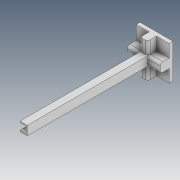
# Autodesk Inventor part: suporte para arma
Saved by Autodesk Inventor 2021 (Build 250183000, 183)
## iProperties
Created: 2020-10-22
Part Number: suporte para arma
Material: Genérico
Document SubType Name: Modeling
Designer: evert
Density: 1 g/cm^3
Appearance: Padrão
Author: evert
Autodesk Inventor part; units mm, degrees
ref_plane "YZ Plane" through (0, 0, 0) normal (1, 0, 0) x (0, 1, 0)
ref_plane "XZ Plane" through (0, 0, 0) normal (0, 1, 0) x (-1, 0, 0)
ref_plane "XY Plane" through (0, 0, 0) normal (0, 0, 1) x (1, 0, 0)
sketch "Esboço1" plane through (0, 0, 0) normal (0, 0, 1) x (1, 0, 0)
  point P0 (0, 0)
sketch "Esboço2" plane through (0, 0, 0) normal (0, 0, 1) x (1, 0, 0)
  line L0 (0, 0) -> (0, 7.2)
  line L1 (0, 7.2) -> (-5.75, 7.2)
  line L2 (-5.75, 7.2) -> (-5.75, 6.2)
  line L3 (-5.75, 6.2) -> (-1, 6.2)
  line L4 (-1, 6.2) -> (-1, 1)
  line L5 (0, 0) -> (-5.75, 0)
  line L6 (-5.75, 0) -> (-5.75, 1)
  line L7 (-5.75, 1) -> (-1, 1)
  dimension "d0" = 7.2
  dimension "d1" = 1
  dimension "d2" = 5.75
  dimension "d3" = 4.75
  dimension "d4" = 5.2
  constraints: 16 end point, 5 perpendicular, 2 horizontal, 1 vertical
  measures "d0" distance of L0.start L0.end
  measures "d1" distance of L1.end L2.end
  measures "d2" distance of L0.end L1.end
  measures "d3" distance of L2.end L3.end
  measures "d4" distance of L3.end L4.end
extrude "Extrusão1" add sketch "Esboço2" along normal blind 105
sketch "Esboço3" plane through (-5.75, 0, 0) normal (0, -1, 0) x (1, 0, 0)
  line L0 (5.75, 0) -> (5.75, 105) projected
  line L1 (5.75, 0) -> (5.75, 10)
  line L2 (5.75, 10) -> (0, 10)
  line L3 (0, 0) -> (0, 105) projected
  line L4 (0, 10) -> (0, 0)
  line L5 (0, 0) -> (5.75, 0) projected
  line L6 (0, 0) -> (5.75, 0)
  dimension "d7" = 10
  constraints: 8 end point, 2 perpendicular, 2 point on line, 1 vertical
  measures "d7" distance of L0.start L1.end
extrude "Extrusão2" add sketch "Esboço3" along normal blind 10
sketch "Esboço4" plane through (0, 0, 105) normal (1, 0, 0) x (0, 0, -1)
  line L0 (105, -10) -> (105, 7.2) projected
  line L1 (105, 0) -> (105, 7.2)
  line L2 (95, 0) -> (95, -10) projected
  line L3 (105, 0) -> (95, 0)
  line L4 (95, 0) -> (95, 7.2)
  line L5 (105, 7.2) -> (0, 7.2) projected
  line L6 (95, 7.2) -> (105, 7.2)
  constraints: 8 end point, 2 perpendicular, 1 collinear, 1 vertical
extrude "Extrusão3" add sketch "Esboço4" along normal blind 10
sketch "Esboço5" plane through (-5.75, 7.2, 105) normal (0, 1, 0) x (1, 0, 0)
  line L0 (0, 105) -> (5.75, 105)
  line L1 (0, 105) -> (15.75, 105) projected
  line L2 (5.75, 105) -> (5.75, 95) projected
  line L3 (5.75, 95) -> (5.75, 105)
  line L4 (5.75, 95) -> (5.75, 0) projected
  line L5 (5.75, 105) -> (5.75, 95)
  line L6 (5.75, 95) -> (0, 95)
  line L7 (0, 105) -> (0, 0) projected
  line L8 (0, 95) -> (0, 105)
  constraints: 10 end point, 4 collinear, 1 perpendicular, 1 point on line
extrude "Extrusão4" add sketch "Esboço5" along normal blind 10
sketch "Esboço6" plane through (0, 7.2, 10) normal (1, 0, 0) x (0, 0, -1)
  line L0 (10, -6.2) -> (10, -17.2) projected
  line L1 (10, -7.2) -> (0, -7.2) projected
  line L2 (10, -17.2) -> (7, -17.2)
  line L3 (7, -17.2) -> (7, -7.2)
  line L4 (7, -7.2) -> (10, -7.2)
  line L5 (10, -7.2) -> (10, -17.2)
  line L6 (10, -1) -> (10, 10) projected
  line L7 (10, 10) -> (0, 10) projected
  line L8 (10, 0) -> (7, 0)
  line L9 (7, 0) -> (7, 10)
  line L10 (7, 10) -> (10, 10)
  line L11 (10, 10) -> (10, 0)
  dimension "d14" = 3
  constraints: 16 end point, 4 parallel, 4 point on line, 2 horizontal, 2 perpendicular
  measures "d14" distance of L3.end L4.end
extrude "Extrusão5" add sketch "Esboço6" along normal blind 10
fillet "Arredondamento1" radius 2 4 edges at (5, 7.2, 10) (0, 12.2, 10) (5, 0, 10) (0, -5, 10)
sketch "Esboço7" plane through (-1, 1, 0) normal (-1, 0, 0) x (0, 0, 1)
  line L0 (10, -1) -> (10, -11) projected
  line L1 (10, 16.2) -> (10, 6.2) projected
  line L2 (10, -1) -> (10, 6.2)
  line L3 (0, 0) -> (0, -11) projected
  line L4 (0, 5.2) -> (105, 5.2) projected
  line L5 (0, 0) -> (10, 0)
  line L6 (10, 0) -> (10, 5.2)
  line L7 (10, 5.2) -> (0, 5.2)
  line L8 (0, 5.2) -> (0, 0)
  point P0 (0, -1)
  constraints: 10 end point, 2 parallel, 2 point on line, 1 collinear, 1 horizontal, 1 perpendicular
extrude "Extrusão6" add sketch "Esboço7" along normal blind 15
sketch "Esboço8" plane through (-5.75, 7.2, 10) normal (-1, 0, 0) x (0, 0, 1)
  line L0 (-10, 10) -> (0, 10) projected
  line L1 (-7, -7.2) -> (-7, -17.2) projected
  line L2 (-10, 10) -> (-7, 10)
  line L3 (-7, 10) -> (-7, -17.2)
  line L4 (-7, -17.2) -> (-10, -17.2)
  line L5 (-10, -17.2) -> (-10, 10)
  point P0 (-10, -7.2)
  constraints: 8 end point, 2 parallel, 1 horizontal, 1 perpendicular
extrude "Extrusão7" add sketch "Esboço8" along normal blind 10.25
fillet "Arredondamento2" radius 2 4 edges at (-5.75, 12.2, 10) (-10.875, 6.2, 10) (-10.875, 1, 10) (-5.75, -5, 10)
